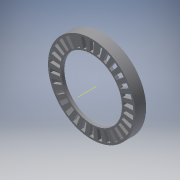
# Autodesk Inventor part: otackomer_new
Saved by Autodesk Inventor 2016 (Build 200138000, 138)
## iProperties
Created: 2015-06-20
Part Number: otackomer_new
Material: Generic
Document SubType Name: Modeling
Designer: Jufo
Density: 1 g/cm^3
Appearance: Default
Author: Jufo
Autodesk Inventor part; units mm, degrees
ref_plane "YZ Plane" through (0, 0, 0) normal (1, 0, 0) x (0, 1, 0)
ref_plane "XZ Plane" through (0, 0, 0) normal (0, 1, 0) x (-1, 0, 0)
ref_plane "XY Plane" through (0, 0, 0) normal (0, 0, 1) x (1, 0, 0)
sketch "Sketch1" plane through (0, 0, 0) normal (0, 1, 0) x (-1, 0, 0)
  circle A0 centre (0, 0) radius 28
  circle A1 centre (0, 0) radius 26.75
  circle A2 centre (0, 0) radius 20.5
  circle A3 centre (0, 0) radius 19.5
  line L0 (0, 20.5) -> (-3, 20.5)
  line L1 (0, 20.5) -> (3, 20.5)
  line L2 (0, 20.5) -> (0, 26.75)
  line L3 (0, 26.75) -> (-4, 26.75)
  line L4 (0, 26.75) -> (4, 26.75)
  line L5 (4, 26.75) -> (3, 20.5)
  line L6 (-4, 26.75) -> (-3, 20.5)
  line L7 (-3, 20.5) -> (-3, 20.2793)
  line L8 (3, 20.5) -> (3, 20.2793)
  arc A4 (3, 20.2793) -> (-3, 20.2793) centre (0, 0) ccw
  arc A5 (3.953, 26.4563) -> (-3.953, 26.4563) centre (0, 0) ccw
  dimension "d0" = 56
  dimension "d1" = 53.5
  dimension "d2" = 41
  dimension "d3" = 39
  dimension "d13" = 8.5
  dimension "d17" = 3
  dimension "d18" = 3
  dimension "d19" = 4
  dimension "d20" = 4
  constraints: 18 end point, 12 point on circle, 6 centre point, 4 coincident, 4 tangent, 3 point on line, 2 horizontal, 2 vertical, 1 parallel, 1 perpendicular
  measures "d0" diameter of A0
  measures "d1" diameter of A1
  measures "d2" diameter of A2
  measures "d3" diameter of A3
  measures "d13" radial gap between concentric circles of A3 A0
  measures "d17" distance of L0.start L1.end
  measures "d18" distance of L0.start L0.end
  measures "d19" distance of L2.end L3.end
  measures "d20" distance of L2.end L4.end
extrude "Extrusion3" add sketch "Sketch1" along normal blind 2 contours A0 | A1 L6 L7 A2 L8 L5 | L5 L1 L2 A1 | A1 L4 L5 | L6 L3 A1 | A1 L2 L0 L6 | L8 A2 L1 | L0 A2 L7 | A2
sketch "Sketch4" plane through (0, 2, 0) normal (0, 1, 0) x (1, 0, 0)
  circle A0 centre (0, 0) radius 28
  circle A1 centre (0, 0) radius 26.75
  circle A2 centre (0, 0) radius 20.5
  circle A3 centre (0, 0) radius 19.5
  line L0 (0, 20.5) -> (-1, 20.5)
  line L1 (0, 20.5) -> (1, 20.5)
  line L2 (0, 20.5) -> (0, 26.75)
  line L3 (0, 26.75) -> (-1.3049, 26.75)
  line L4 (0, 26.75) -> (1.3049, 26.75)
  line L5 (1.3049, 26.75) -> (1, 20.5)
  line L6 (-1.3049, 26.75) -> (-1, 20.5)
  line L7 (-1, 20.5) -> (-1, 20.4756)
  line L8 (1, 20.5) -> (1, 20.4756)
  arc A4 (1, 20.4756) -> (-1, 20.4756) centre (0, 0) ccw
  arc A5 (1.3033, 26.7182) -> (-1.3033, 26.7182) centre (0, 0) ccw
  dimension "d23" = 56
  dimension "d24" = 53.5
  dimension "d25" = 41
  dimension "d26" = 39
  dimension "d27" = 8.5
  dimension "d28" = 1
  dimension "d29" = 1
  dimension "d30" = 1.3049
  dimension "d31" = 1.3049
  constraints: 18 end point, 12 point on circle, 6 centre point, 4 coincident, 4 tangent, 3 point on line, 2 horizontal, 2 vertical, 1 parallel, 1 perpendicular
  measures "d23" diameter of A0
  measures "d24" diameter of A1
  measures "d25" diameter of A2
  measures "d26" diameter of A3
  measures "d27" radial gap between concentric circles of A3 A0
  measures "d28" distance of L0.start L1.end
  measures "d29" distance of L0.start L0.end
  measures "d30" distance of L2.end L3.end
  measures "d31" distance of L2.end L4.end
extrude "Extrusion4" cut sketch "Sketch4" against normal blind 10 contours L5 L1 L2 A1 | A1 L2 L0 L6 | L8 A2 L1 | L0 A2 L7
pattern_circular "Circular Pattern2" count 30 over 360 about axis through (0, 2, 0) along (0, -1, 0) of "Extrusion4"
sketch "Sketch5" plane through (0, 2, 0) normal (0, 1, 0) x (1, 0, 0)
  circle A0 centre (0, 0) radius 28
  line L0 (-1, 20.5) -> (-1.3033, 26.7182) projected
  circle A1 centre (0, 0) radius 26.75
  constraints: 2 coincident, 1 centre point, 3 other
extrude "Extrusion5" add sketch "Sketch5" along normal blind 5
equation "\"d29\" = d28"
equation "\"d30\" = d31"
body "Solid2"
